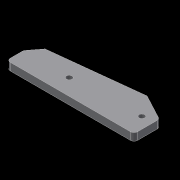
# Autodesk Inventor part: SpineNeckLinkConnector
Saved by Autodesk Inventor 2015 (Build 190159000, 159)
## iProperties
Created: 2015-01-13
Part Number: SpineNeckLinkConnector
Material: Generic
Document SubType Name: Modeling
Designer: Inventor
Mass: 4.8787 g
Surface Area: 33.6096 cm^2
Volume: 4.8787 cm^3
Density: 1 g/cm^3
Appearance: Default
RuleStatus: InUse
BeforeDocSave0: UpdateBoundingBox
CX: 74.00 mm
CY: 21.00 mm
CZ: 4.00 mm
Author: Inventor
Autodesk Inventor part; units mm, degrees
ref_plane "YZ Plane" through (0, 0, 0) normal (1, 0, 0) x (0, 1, 0)
ref_plane "XZ Plane" through (0, 0, 0) normal (0, 1, 0) x (-1, 0, 0)
ref_plane "XY Plane" through (0, 0, 0) normal (0, 0, 1) x (1, 0, 0)
sketch "Body" plane through (0, 0, 0) normal (0, 0, 1) x (1, 0, 0)
  line L0 (0, 0) -> (60, 0) construction
  line L1 (-7, 2) -> (-2, 8.5)
  line L2 (-2, 8.5) -> (53, 14)
  line L3 (53, 14) -> (67, 6.5)
  line L4 (67, 6.5) -> (67, -7)
  line L5 (67, -7) -> (-7, -7)
  line L6 (-7, -7) -> (-7, 2)
  dimension "d1" = 60
  dimension "d2" = 7
  dimension "d4" = 7
  dimension "d5" = 7
  dimension "d6" = 14
  dimension "d8" = 13.5
  dimension "d9" = 9
  dimension "d13" = 8.5
  dimension "d14" = 5
  dimension "d15" = 14
  constraints: 14 end point, 2 perpendicular, 1 coincident, 1 horizontal
  measures "d1" distance of L0.start L0.end
  measures "d2" distance between parallel lines of L5 L0
  measures "d4" distance from line of point (0, 0) L6
  measures "d5" distance from line of L4 L0.end
  measures "d6" horizontal distance of L2.end L3.end
  measures "d8" distance of L3.end L4.end
  measures "d9" distance of L5.end L1.start
  measures "d13" vertical distance of L1.end point (0, 0)
  measures "d14" horizontal distance of L1.start L1.end
  measures "d15" distance from line of L2.end L0
extrude "BodyFeature" add sketch "Body" along normal blind 4
fillet "FilletsFeature" radius 2 4 edges at (-7, -7, 2) (67, -7, 2) (-7, 2, 2) (67, 6.5, 2)
sketch "MountHoles" plane through (0, 0, 4) normal (0, 0, 1) x (1, 0, 0)
  circle A0 centre (1.2887, 0.4289) radius 3.25 projected
  circle A1 centre (25.2886, 0.4803) radius 3.25 projected
  circle A2 centre (58.3386, 1.9174) radius 3.25 projected
hole "MountHolesFeature" at (1.2887, 0.4289, 4) at (25.2886, 0.4803, 4) at (58.3386, 1.9174, 4) direction (0, 0, -1) diameter 6 end through all
